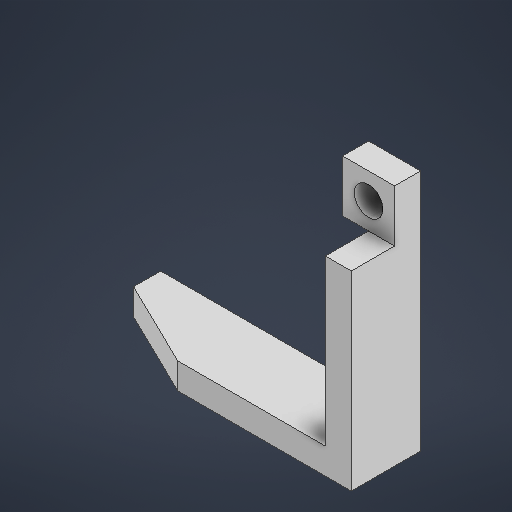
# Autodesk Inventor part: rightfrontwall
Saved by Autodesk Inventor 2026.2 (Build 302298010, 298A)
## iProperties
Created: 2026-09-21
Part Number: rightfrontwall
Material: Generic
Document SubType Name: Modeling
Designer: karol
Density: 1 g/cm^3
Appearance: Default
Author: karol
Autodesk Inventor part; units mm, degrees
ref_plane "YZ Plane" through (0, 0, 0) normal (1, 0, 0) x (0, 1, 0)
ref_plane "XZ Plane" through (0, 0, 0) normal (0, 1, 0) x (-1, 0, 0)
ref_plane "XY Plane" through (0, 0, 0) normal (0, 0, 1) x (1, 0, 0)
sketch "Sketch1" plane through (0, 0, 0) normal (0, 0, 1) x (1, 0, 0)
  line L0 (-58, -60) -> (-60, -60) projected
  line L1 (-60, -60) -> (-60, -39.5) projected
  line L2 (-60, -39.5) -> (-58, -39.5) projected
  line L3 (-58, -39.5) -> (-58, -60) projected
  line L4 (49.6, 30) -> (51.6, 30) projected
  line L5 (51.6, 30) -> (51.6, 9.5) projected
  line L6 (51.6, 9.5) -> (49.6, 9.5) projected
  line L7 (49.6, 9.5) -> (49.6, 30) projected
  line L8 (-58, 39.5) -> (-60, 39.5) projected
  line L9 (-60, 39.5) -> (-60, 60) projected
  line L10 (-60, 60) -> (-58, 60) projected
  line L11 (-58, 60) -> (-58, 39.5) projected
  line L12 (-21.6, -39.5) -> (-19.6, -39.5) projected
  line L13 (-19.6, -39.5) -> (-19.6, -60) projected
  line L14 (-19.6, -60) -> (-21.6, -60) projected
  line L15 (-21.6, -60) -> (-21.6, -39.5) projected
  line L16 (51.6, -30) -> (49.6, -30) projected
  line L17 (49.6, -30) -> (49.6, -9.5) projected
  line L18 (49.6, -9.5) -> (51.6, -9.5) projected
  line L19 (51.6, -9.5) -> (51.6, -30) projected
  line L20 (-21.6, 60) -> (-19.6, 60) projected
  line L21 (-19.6, 60) -> (-19.6, 39.5) projected
  line L22 (-19.6, 39.5) -> (-21.6, 39.5) projected
  line L23 (-21.6, 39.5) -> (-21.6, 60) projected
  line L24 (90, -35) -> (90, 35) projected
  line L25 (90, 35) -> (49.6, 35) projected
  line L26 (49.6, 35) -> (49.6, 60) projected
  line L27 (49.6, 60) -> (90, 60) projected
  line L28 (90, 60) -> (90, 90) projected
  line L29 (90, 90) -> (-19.6, 90) projected
  line L30 (-19.6, 90) -> (-19.6, 65) projected
  line L31 (-19.6, 65) -> (-60, 65) projected
  line L32 (-60, 65) -> (-60, 90) projected
  line L33 (-60, 90) -> (-90, 90) projected
  line L34 (-90, 90) -> (-90, -90) projected
  line L35 (-90, -90) -> (-60, -90) projected
  line L36 (-60, -90) -> (-60, -65) projected
  line L37 (-60, -65) -> (-19.6, -65) projected
  line L38 (-19.6, -65) -> (-19.6, -90) projected
  line L39 (-19.6, -90) -> (90, -90) projected
  line L40 (90, -90) -> (90, -60) projected
  line L41 (90, -60) -> (49.6, -60) projected
  line L42 (49.6, -60) -> (49.6, -35) projected
  line L43 (49.6, -35) -> (90, -35) projected
  line L44 (86, -32) -> (73.8, -32) projected
  line L45 (73.8, -32) -> (73.8, -7.5) projected
  line L46 (73.8, -7.5) -> (86, -7.5) projected
  line L47 (86, -7.5) -> (86, -32) projected
  line L48 (65.8, -32) -> (53.6, -32) projected
  line L49 (53.6, -32) -> (53.6, -7.5) projected
  line L50 (53.6, -7.5) -> (65.8, -7.5) projected
  line L51 (65.8, -7.5) -> (65.8, -32) projected
  line L52 (86, -86) -> (70.6, -86) projected
  line L53 (70.6, -86) -> (70.6, -69.8) projected
  line L54 (70.6, -69.8) -> (86, -69.8) projected
  line L55 (86, -69.8) -> (86, -86) projected
  line L56 (86, 86) -> (86, 69.8) projected
  line L57 (86, 69.8) -> (70.6, 69.8) projected
  line L58 (70.6, 69.8) -> (70.6, 86) projected
  line L59 (70.6, 86) -> (86, 86) projected
  line L60 (73.8, 32) -> (86, 32) projected
  line L61 (86, 32) -> (86, 7.5) projected
  line L62 (86, 7.5) -> (73.8, 7.5) projected
  line L63 (73.8, 7.5) -> (73.8, 32) projected
  line L64 (65.8, 32) -> (65.8, 7.5) projected
  line L65 (65.8, 7.5) -> (53.6, 7.5) projected
  line L66 (53.6, 7.5) -> (53.6, 32) projected
  line L67 (53.6, 32) -> (65.8, 32) projected
  line L68 (-69.6, -87) -> (-85, -87) projected
  line L69 (-85, -87) -> (-85, -70.8) projected
  line L70 (-85, -70.8) -> (-69.6, -70.8) projected
  line L71 (-69.6, -70.8) -> (-69.6, -87) projected
  line L72 (-56, -62) -> (-56, -37.5) projected
  line L73 (-56, -37.5) -> (-43.8, -37.5) projected
  line L74 (-43.8, -37.5) -> (-43.8, -62) projected
  line L75 (-43.8, -62) -> (-56, -62) projected
  line L76 (-56, 62) -> (-43.8, 62) projected
  line L77 (-43.8, 62) -> (-43.8, 37.5) projected
  line L78 (-43.8, 37.5) -> (-56, 37.5) projected
  line L79 (-56, 37.5) -> (-56, 62) projected
  line L80 (-23.6, 62) -> (-23.6, 37.5) projected
  line L81 (-23.6, 37.5) -> (-35.8, 37.5) projected
  line L82 (-35.8, 37.5) -> (-35.8, 62) projected
  line L83 (-35.8, 62) -> (-23.6, 62) projected
  line L84 (-23.6, -62) -> (-35.8, -62) projected
  line L85 (-35.8, -62) -> (-35.8, -37.5) projected
  line L86 (-35.8, -37.5) -> (-23.6, -37.5) projected
  line L87 (-23.6, -37.5) -> (-23.6, -62) projected
  line L88 (-85, 87) -> (-69.6, 87) projected
  line L89 (-69.6, 87) -> (-69.6, 70.8) projected
  line L90 (-69.6, 70.8) -> (-85, 70.8) projected
  line L91 (-85, 70.8) -> (-85, 87) projected
  line L92 (-13.6, -62) -> (-66, -62) projected
  line L93 (-66, -62) -> (-66, -68) projected
  line L94 (-66, -68) -> (-60, -68) projected
  line L95 (-60, -68) -> (-60, -65) projected
  line L96 (-60, -65) -> (-19.6, -65) projected
  line L97 (-19.6, -65) -> (-19.6, -68) projected
  line L98 (-19.6, -68) -> (-13.6, -68) projected
  line L99 (-13.6, -68) -> (-13.6, -62) projected
  line L100 (-90, -90) -> (-60, -90)
  line L101 (-60, -90) -> (-60, -87)
  line L102 (-60, -87) -> (-90, -87)
  line L103 (-90, -87) -> (-90, -90)
  line L104 (-60, -87) -> (-63, -87)
  line L105 (-63, -87) -> (-63, -68)
  line L106 (-63, -68) -> (-60, -68)
  line L107 (-60, -68) -> (-60, -87)
  line L108 (-60, -68) -> (-66, -68)
  line L109 (-66, -68) -> (-66, -62)
  line L110 (-66, -62) -> (-60, -62)
  line L111 (-60, -62) -> (-60, -68)
  circle A0 centre (-63, -65) radius 1.5 projected
  circle A1 centre (-16.6, -87) radius 1.5 projected
  circle A2 centre (49.6, -87) radius 1.5 projected
  circle A3 centre (46.6, -60) radius 1.5 projected
  circle A4 centre (87, -63) radius 1.5 projected
  circle A5 centre (46.6, -32) radius 1.5 projected
  circle A6 centre (46.6, 32) radius 1.5 projected
  circle A7 centre (87, 63) radius 1.5 projected
  circle A8 centre (46.6, 60) radius 1.5 projected
  circle A9 centre (49.6, 87) radius 1.5 projected
  circle A10 centre (-16.6, 87) radius 1.5 projected
  circle A11 centre (-16.6, 65) radius 1.5 projected
  circle A12 centre (-63, 65) radius 1.5 projected
  point P0 (0, 0)
  dimension "d0" = 3
  constraints: 24 end point, 6 parallel, 3 horizontal, 3 perpendicular, 2 point on line, 1 midpoint
  measures "d0" distance of L105.end L106.end
extrude "Extrusion1" add sketch "Sketch1" along normal blind 8 contours L36 L102 L105 L94 | L36 L35 L34 L102 L68
ref_plane "Work Plane1" through (0, 0, 0) normal (0, 0, 1) x (1, 0, 0)
sketch "Sketch2" plane through (0, 0, 0) normal (0, 0, 1) x (1, 0, 0)
  line L0 (-13.6, -62) -> (-66, -62) projected
  line L1 (-66, -62) -> (-66, -68) projected
  line L2 (-66, -68) -> (-60, -68) projected
  line L3 (-60, -68) -> (-60, -65) projected
  line L4 (-60, -65) -> (-19.6, -65) projected
  line L5 (-19.6, -65) -> (-19.6, -68) projected
  line L6 (-19.6, -68) -> (-13.6, -68) projected
  line L7 (-13.6, -68) -> (-13.6, -62) projected
  circle A0 centre (-63, -65) radius 2 projected
  line L8 (-60, -90) -> (-60, -68) projected
  line L9 (-60, -68) -> (-66, -68)
  line L10 (-66, -68) -> (-66, -62)
  line L11 (-66, -62) -> (-60, -62)
  line L12 (-60, -62) -> (-60, -68)
  circle A1 centre (-63, -65) radius 1.65
  point P0 (0, 0)
  dimension "d3" = 3.3
  constraints: 8 end point, 2 parallel, 1 centre point, 1 coincident, 1 horizontal, 1 perpendicular
  measures "d3" diameter of A1
extrude "Extrusion2" add sketch "Sketch2" along normal blind 3 contours L12 L3 L2 L1 L0 | A0
sketch "Sketch3" plane through (-90, -90, 0) normal (0, -1, 0) x (1, 0, 0)
  line L0 (0, 0) -> (0, 8) projected
  line L1 (0, 3.137) -> (9.9706, 8)
  line L2 (0, 3.137) -> (11.0933, 3.137) construction
  line L3 (0, 8) -> (30, 8) projected
  point P0 (90, 0)
  dimension "d7" = 26
  dimension "d8" = 3.137
  constraints: 4 end point, 2 point on line, 1 equal length, 1 horizontal
  measures "d7" angle of L2 L1
  measures "d8" distance of L1.start L0.start
extrude "Extrusion3" cut sketch "Sketch3" against normal blind 3
body "Solid1"
